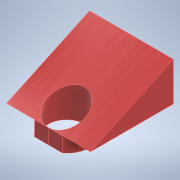
# Autodesk Inventor part: bottomAttachementForPvcPipe
Saved by Autodesk Inventor 2022.2 (Build 262287000, 287)
## iProperties
Created: 2021-10-20
Part Number: bottomAttachementForPvcPipe
Material: PC/ABS Plastic
Document SubType Name: Modeling
Designer: robst
Density: 0.357273 g/cm^3
Appearance: Red
Author: robst
Autodesk Inventor part; units mm, degrees
ref_plane "YZ Plane" through (0, 0, 0) normal (1, 0, 0) x (0, 1, 0)
ref_plane "XZ Plane" through (0, 0, 0) normal (0, 1, 0) x (-1, 0, 0)
ref_plane "XY Plane" through (0, 0, 0) normal (0, 0, 1) x (1, 0, 0)
sketch "Sketch65" plane through (0, 0, 0) normal (1, 0, 0) x (0, 1, 0)
  line L0 (0, 0) -> (64.407, -138.1213)
  line L1 (64.407, -138.1213) -> (0, -138.1213)
  line L2 (0, -138.1213) -> (0, 0)
  dimension "d335" = 25
  dimension "d349" = 152.4
  constraints: 6 end point, 1 horizontal, 1 perpendicular
  measures "d335" angle of L0 L2
  measures "d349" distance of L0.start L0.end
extrude "Extrusion34" add sketch "Sketch65" along normal mid plane 139.7
sketch "Sketch67" plane through (-69.85, 0, -138.1213) normal (0, -1, 0) x (1, 0, 0)
  line L0 (69.85, 138.1213) -> (69.85, 0) construction
  line L1 (0, 0) -> (139.7, 0) construction
  line L2 (0, 138.1213) -> (139.7, 138.1213) projected
  line L3 (139.7, 138.1213) -> (139.7, 0) projected
  line L4 (0, 0) -> (0, 138.1213) projected
  circle A0 centre (69.85, 107.9588) radius 30.1625
  arc A1 (46.4705, 138.1213) -> (93.2295, 138.1213) centre (69.85, 107.9588) ccw
  line L5 (93.2295, 138.1213) -> (69.85, 138.1213)
  line L6 (69.85, 138.1213) -> (46.4705, 138.1213)
  circle A2 centre (69.85, 107.9588) radius 22.1625
  dimension "d338" = 60.325
  dimension "d339" = 8
  dimension "d344" = 8
  constraints: 6 end point, 3 centre point, 3 point on line, 2 coincident, 2 collinear, 2 point on circle, 2 tangent, 1 midpoint
  measures "d338" diameter of A0
  measures "d339" radial gap between concentric circles of A1 A0
  measures "d344" radial gap between concentric circles of A0 A2
extrude "Extrusion37" cut sketch "Sketch67" against normal through all contours A0 | A2
extrude "Extrusion38" add sketch "Sketch67" along normal blind 25 contours L2 A1
equation "\"wallThickness\" = 8"
equation "\"twoByFourWidth\" = 40.64"
equation "\"twoByFourDepth\" = 84.1375"
equation "\"azimuth\" = 55deg"
equation "\"elevationOfTwoByFour\" = 20deg"
equation "\"depthOfExtrusionForMatingToLowerHalf\" = 12.5"
equation "\"depthForWasherForMatingToCase\" = 14"
equation "\"pvc2InchPipeInsideDiameter\" = 52.5018"
equation "\"pvc2InchPipeOutsideDiameter\" = 60.325"
equation "\"pvcPipeInsertDepth\" = 25"
equation "\"outsideDiameterOfPipe\" = 88.9"
equation "\"insideDiameterOfPipe\" = 76.2"
equation "\"outsideDiameterOfPart\" = 114.3"
equation "\"pvc3InchPipeOutsideDiameter\" = 88.9"
body "Solid4"
body "Solid6"
